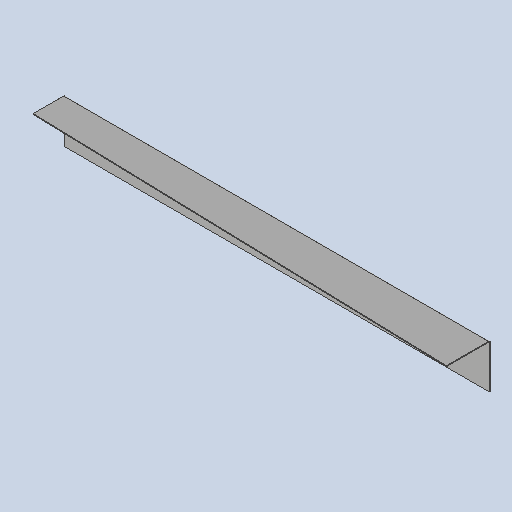
# Autodesk Inventor part: NDV-2102 Collector top 01
Saved by Autodesk Inventor 2026.2 (Build 302298000, 298)
## iProperties
Created: 2024-12-09
Part Number: NDV-2102 Collector top 01
Material: Stainless Steel
Document SubType Name: Sheet Metal
Designer: admin
Mass: 793.765 g
Surface Area: 1023.32 cm^2
Volume: 99.2206 cm^3
Density: 8 g/cm^3
Flat Pattern Width: 21.5202 cm
Flat Pattern Length: 105 cm
Flat Pattern Area: 2259.62 cm^2
Sheet Metal Rule: AISI304 2mm Die16
Sheet Metal Width: 215,202 mm
Sheet Metal Length: 1050,000 mm
Sheet Metal Area: 225962,090 mm^2
Appearance: Default
Stock Number: Коллектор верх
Main_way_hight: 100,000 mm
Main_way_lenth: 410,000 mm
Author: user
Autodesk Inventor part; units mm, degrees
ref_plane "YZ Plane" through (0, 0, 0) normal (1, 0, 0) x (0, 1, 0)
ref_plane "XZ Plane" through (0, 0, 0) normal (0, 1, 0) x (-1, 0, 0)
ref_plane "XY Plane" through (0, 0, 0) normal (0, 0, 1) x (1, 0, 0)
sketch "Sketch1" plane through (0, 0, 0) normal (0, 0, 1) x (1, 0, 0)
  line L0 (0, 0) -> (-1050, 0)
  line L1 (0, -109) -> (0, 0)
  line L2 (-1050, 0) -> (-1050, -80)
  line L3 (-1050, -80) -> (0, -109)
  point P0 (0, -54.5)
  dimension "d32" = 109
  dimension "d60" = 80
  dimension "d61" = 1050
  measures "d32" distance of L1.start L0.start
  measures "d60" distance of L0.end L2.end
  measures "d61" distance between parallel lines of L1 L2
extrude "Plate1" add sketch "Sketch1" along normal blind 2
sketch "Sketch8" plane through (0, 0, 2) normal (0, 0, 1) x (1, 0, 0)
  line L0 (-24.75, -58.25) -> (-65.25, -58.25)
  line L1 (-65.25, -58.25) -> (-65.25, -17.75)
  line L2 (-65.25, -17.75) -> (-24.75, -17.75)
  line L3 (-24.75, -17.75) -> (-24.75, -58.25)
  line L4 (-24.75, -58.25) -> (-65.25, -17.75) construction
  line L5 (-65.25, -58.25) -> (-24.75, -17.75) construction
  circle A0 centre (-22, -61) radius 2.5
  circle A1 centre (-68, -61) radius 2.5
  circle A2 centre (-68, -15) radius 2.5
  circle A3 centre (-22, -15) radius 2.5
  line L6 (0, 0) -> (0, -109) projected
  line L7 (-1050, 0) -> (0, 0) projected
  line L8 (-65.25, -58.25) -> (-68, -61) construction
  line L9 (-68, -15) -> (-22, -15) construction
  line L10 (-22, -15) -> (-22, -61) construction
  line L11 (-22, -61) -> (-68, -61) construction
  line L12 (-68, -61) -> (-68, -15) construction
  point P0 (-45, -38)
  dimension "d51" = 40.5
  dimension "d52" = 40.5
  dimension "d53" = 5
  dimension "d72" = 45
  dimension "d78" = 46
  dimension "d79" = 15
  constraints: 22 end point, 4 centre point, 4 parallel, 4 point on line, 3 equal radius, 2 horizontal, 2 midpoint, 2 perpendicular
  measures "d51" distance of L0.start L0.end
  measures "d52" distance of L0.end L1.end
  measures "d53" diameter of A0
  measures "d72" distance from line of L6 point (-45, -38)
  measures "d78" distance of L8.end L9.start
  measures "d79" distance between parallel lines of L9 L7
cut "Cut3" [suppressed]
pattern_linear "Rectangular Pattern1" [suppressed]
sketch "Sketch9" plane through (0, -2, 2) normal (0, 1, 0) x (-1, 0, 0)
  line L0 (1050, 0) -> (0, 0)
  line L1 (0, 0) -> (0, -110)
  line L2 (0, -110) -> (1050, -110)
  line L3 (1050, -110) -> (1050, 0)
  constraints: 6 end point, 1 horizontal, 1 perpendicular, 1 vertical
edge flange "Flange3" height 110 angle 90 thickness 2 bend radius 2.75 thickness toward (0, 1, 0) relief round relief width 2 relief depth 1 edges at (-525, 0, 0) wall of the first edge with corners at (-1050, -2, 2) (0, -2, 2) (0, -2, -108) (-1050, -2, -108)
bend "Bend3"
corner "Corner3"
derived "NDV-0010 Parameters 01.ipt"
equation "\"d51\" = d52"
equation "\"d55\" = Thickness"
equation "\"d2\" = Thickness"
equation "\"d62\" = BendReliefWidth"
equation "\"d63\" = BendReliefDepth"
equation "\"d64\" = MinimumRemnant"
equation "\"d65\" = TransitionRadius"
equation "\"d68\" = BendRadius"
equation "\"d69\" = CornerReliefSize"
equation "\"d70\" = GapSize"
equation "\"d71\" = JacobiRadiusSize"
equation "\"BendReliefWidth\" = Thickness"
equation "\"BendReliefDepth\" = 0.5 * Thickness"
equation "\"CornerReliefSize\" = 4 * Thickness"
equation "\"MinimumRemnant\" = 2 * Thickness"
equation "\"TransitionRadius\" = BendRadius"
equation "\"JacobiRadiusSize\" = BendRadius"
equation "\"GapSize\" = Thickness"
equation "\"Thickness\" = 2"
equation "\"BendRadius\" = 2.75"
body "Solid1"
